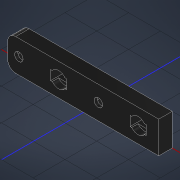
# Autodesk Inventor part: Door_Basis
Saved by Autodesk Inventor 2022.2 (Build 262287010, 287A)
## iProperties
Created: 2022-01-24
Part Number: Door_Basis
Material: ABS-Kunststoff
Document SubType Name: Modeling
Designer: sleib
Density: 1.06 g/cm^3
Appearance: Glatt - Schwarz
Author: sleib
Autodesk Inventor part; units mm, degrees
ref_plane "YZ Plane" through (0, 0, 0) normal (1, 0, 0) x (0, 1, 0)
ref_plane "XZ Plane" through (0, 0, 0) normal (0, 1, 0) x (-1, 0, 0)
ref_plane "XY Plane" through (0, 0, 0) normal (0, 0, 1) x (1, 0, 0)
sketch "Skizze1" plane through (0, 0, 0) normal (0, 0, 1) x (1, 0, 0)
  line L0 (47.5, -10) -> (-47.5, -10)
  line L1 (-47.5, -10) -> (-47.5, 10)
  line L2 (-47.5, 10) -> (47.5, 10)
  line L3 (47.5, 10) -> (47.5, -10)
  line L4 (47.5, -10) -> (-47.5, 10) construction
  line L5 (-47.5, -10) -> (47.5, 10) construction
  circle A0 centre (-40.5, 0) radius 2.65
  circle A1 centre (9.5, 0) radius 2.65
  line L6 (-44.75, -2.4537) -> (-44.75, 2.4537)
  line L7 (-44.75, 2.4537) -> (-40.5, 4.9075)
  line L8 (-40.5, 4.9075) -> (-36.25, 2.4537)
  line L9 (-36.25, 2.4537) -> (-36.25, -2.4537)
  line L10 (-36.25, -2.4537) -> (-40.5, -4.9075)
  line L11 (-40.5, -4.9075) -> (-44.75, -2.4537)
  line L12 (5.25, -2.4537) -> (5.25, 2.4537)
  line L13 (5.25, 2.4537) -> (9.5, 4.9075)
  line L14 (9.5, 4.9075) -> (13.75, 2.4537)
  line L15 (13.75, 2.4537) -> (13.75, -2.4537)
  line L16 (13.75, -2.4537) -> (9.5, -4.9075)
  line L17 (9.5, -4.9075) -> (5.25, -2.4537)
  point P0 (0, 0)
  point P1 (0, 0)
  point P2 (0, 0)
  point P3 (-2.125, 0)
  point P4 (-2.125, 0)
  point P5 (-2.125, 0)
  dimension "d0" = 20
  dimension "d2" = 5.3
  dimension "d3" = 5.3
  dimension "d4" = 50
  dimension "d13" = 38
  dimension "d26" = 8.5
  dimension "d27" = 8.5
  dimension "d42" = 7
  constraints: 36 end point, 4 midpoint, 3 horizontal alignment, 2 centre point, 2 coincident, 2 parallel, 2 vertical, 1 horizontal, 1 perpendicular, 26 other
  measures "d0" distance of L0.end L1.end
  measures "d2" diameter of A0
  measures "d3" diameter of A1
  measures "d4" distance of A1.centre A0.centre
  measures "d13" distance from line of L3 A1.centre
  measures "d26" distance between parallel lines of L9 L6
  measures "d27" distance between parallel lines of L15 L12
  measures "d42" distance from line of L1 A0.centre
extrude "Extrusion1" add sketch "Skizze1" along normal blind 8.5 contours L0 L1 L2 L3 | L6 L7 L8 L9 L10 L11 | L12 L13 L14 L15 L16 L17
extrude "Extrusion2" cut sketch "Skizze1" along normal blind 6.5 contours A1 | L6 L7 L8 L9 L10 L11 | L12 L13 L14 L15 L16 L17
sketch "Skizze2" plane through (0, 0, 8.5) normal (0, 0, 1) x (1, 0, 0)
  line L0 (-47.5, -10) -> (47.5, -10) projected
  line L1 (47.5, -10) -> (47.5, 10) projected
  line L2 (47.5, 10) -> (-47.5, 10) projected
  line L3 (-47.5, 10) -> (-47.5, -10) projected
  line L4 (-47.5, 10) -> (-47.5, -10) projected
  line L5 (-47.5, 0) -> (47.5, 0) construction
  line L6 (47.5, -10) -> (47.5, 10) projected
  point P0 (0, 0)
  point P1 (-15.5, 0)
  point P2 (34.5, 0)
  constraints: 2 end point, 2 midpoint, 2 point on line
hole "Bohrung1" at (-15.5, 0, 8.5) at (34.5, 0, 8.5) direction (0, 0, -1) diameter 5.3 end through all counterbore diameter 10 counterbore depth 4 clearance for "Inbusschraube DIN EN ISO 4762" size "M5" standard "DIN"
fillet "Rundung1" radius 5 2 edges at (-47.5, -10, 4.25) (-47.5, 10, 4.25)
sketch "Skizze3" plane through (0, 0, 8.5) normal (0, 0, 1) x (1, 0, 0)
  line L0 (39.5, 3) -> (29.5, 3)
  line L1 (29.5, 3) -> (29.5, -3)
  line L2 (29.5, -3) -> (39.5, -3)
  line L3 (39.5, -3) -> (39.5, 3)
  circle A0 centre (34.5, 0) radius 2.65 projected
  line L4 (39.5, 3) -> (29.5, -3) construction
  line L5 (29.5, 3) -> (39.5, -3) construction
  circle A1 centre (-15.5, 0) radius 2.65 projected
  line L6 (-10.5, 3) -> (-20.5, 3)
  line L7 (-20.5, 3) -> (-20.5, -3)
  line L8 (-20.5, -3) -> (-10.5, -3)
  line L9 (-10.5, -3) -> (-10.5, 3)
  line L10 (-10.5, 3) -> (-20.5, -3) construction
  line L11 (-20.5, 3) -> (-10.5, -3) construction
  point P0 (0, 0)
  dimension "d51" = 6
  dimension "d52" = 10
  constraints: 24 end point, 4 midpoint, 4 parallel, 2 equal length, 2 horizontal, 2 perpendicular
  measures "d51" distance between parallel lines of L0 L2
  measures "d52" distance between parallel lines of L1 L3
extrude "Extrusion4" cut sketch "Skizze3" against normal through all
equation "\"d3\" = d2"
equation "\"d27\" = d26"
